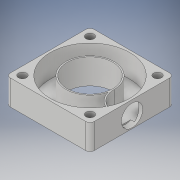
# Autodesk Inventor part: base3
Saved by Autodesk Inventor 2019 (Build 230136000, 136)
## iProperties
Created: 2020-10-29
Part Number: base3
Material: Genérico
Document SubType Name: Modeling
Designer: Juan M. Casillas
Density: 1 g/cm^3
Appearance: Valor por defecto
Author: Juan M. Casillas
## iProperties of the stored document base3_3DPrint.ipt
Created: 2020-10-29
Part Number: base3_3DPrint
Material: Genérico
Document SubType Name: Modeling
Designer: Juan M. Casillas
Density: 1 g/cm^3
Appearance: Valor por defecto
Author: Juan M. Casillas
Autodesk Inventor part; units mm, degrees
ref_plane "YZ Plane" through (0, 0, 0) normal (1, 0, 0) x (0, 1, 0)
ref_plane "XZ Plane" through (0, 0, 0) normal (0, 1, 0) x (-1, 0, 0)
ref_plane "XY Plane" through (0, 0, 0) normal (0, 0, 1) x (1, 0, 0)
sketch "Sketch1" plane through (0, 0, 0) normal (0, 1, 0) x (-1, 0, 0)
  line L0 (18, 20) -> (-18, 20)
  line L1 (-20, 18) -> (-20, -18)
  line L2 (-18, -20) -> (18, -20)
  line L3 (20, -18) -> (20, 18)
  line L4 (20, 20) -> (-20, -20) construction
  line L5 (-20, 20) -> (20, -20) construction
  circle A0 centre (0, 0) radius 11.5
  circle A1 centre (0, 0) radius 18.945
  arc A2 (20, 18) -> (18, 20) centre (18, 18) ccw
  arc A3 (18, -20) -> (20, -18) centre (18, -18) ccw
  arc A4 (-20, -18) -> (-18, -20) centre (-18, -18) ccw
  arc A5 (-18, 20) -> (-20, 18) centre (-18, 18) ccw
  dimension "d0" = 40
  dimension "d1" = 40
  dimension "d2" = 23
  dimension "d3" = 37.89
  dimension "d4" = 2
  constraints: 12 end point, 8 point on circle, 8 point on line, 8 tangent, 6 centre point, 3 equal radius, 2 coincident, 2 midpoint, 2 parallel, 1 horizontal, 1 perpendicular
  measures "d0" distance of L5.end L4.end
  measures "d1" distance of L4.end L5.start
  measures "d2" diameter of A0
  measures "d3" diameter of A1
  measures "d4" radius of A2
extrude "Extrusion1" add sketch "Sketch1" along normal blind 11
sketch "Sketch2" plane through (0, 0, 0) normal (0, -1, 0) x (1, 0, 0)
  line L0 (-20, -18) -> (-20, 18) projected
  arc A0 (-18, 20) -> (-20, 18) centre (-18, 18) ccw projected
  line L1 (-18, 20) -> (18, 20) projected
  arc A1 (20, 18) -> (18, 20) centre (18, 18) ccw projected
  line L2 (20, 18) -> (20, -18) projected
  arc A2 (18, -20) -> (20, -18) centre (18, -18) ccw projected
  line L3 (18, -20) -> (-18, -20) projected
  arc A3 (-20, -18) -> (-18, -20) centre (-18, -18) ccw projected
  point P0 (0, 0)
extrude "Extrusion2" add sketch "Sketch2" against normal blind 1
sketch "Sketch3" plane through (0, 11, 0) normal (0, 1, 0) x (1, 0, 0)
  circle A0 centre (0, 0) radius 11.5 projected
  circle A1 centre (0, 0) radius 10.9
  dimension "d9" = 0.6
  constraints: 1 centre point
  measures "d9" radial gap between concentric circles of A0 A1
extrude "Extrusion3" cut sketch "Sketch3" against normal through all contours A1
sketch "Sketch4" plane through (0, 11, 0) normal (0, 1, 0) x (1, 0, 0)
  circle A0 centre (0, 0) radius 18.945 construction
  line L0 (-18, -20) -> (18, -20) construction
  arc A1 (18, -20) -> (20, -18) centre (18, -18) ccw construction
  line L1 (20, -18) -> (20, 18) construction
  arc A2 (20, 18) -> (18, 20) centre (18, 18) ccw construction
  line L2 (18, 20) -> (-18, 20) construction
  arc A3 (-18, 20) -> (-20, 18) centre (-18, 18) ccw construction
  line L3 (-20, 18) -> (-20, -18) construction
  arc A4 (-20, -18) -> (-18, -20) centre (-18, -18) ccw construction
  line L4 (-16.1, -16.1) -> (16.1, -16.1) construction
  line L5 (16.1, -16.1) -> (16.1, 16.1) construction
  line L6 (16.1, 16.1) -> (-16.1, 16.1) construction
  line L7 (-16.1, 16.1) -> (-16.1, -16.1) construction
  line L8 (-16.1, -16.1) -> (16.1, 16.1) construction
  line L9 (16.1, -16.1) -> (-16.1, 16.1) construction
  point P0 (0, 0)
  dimension "d12" = 32.2
  dimension "d13" = 32.2
  constraints: 12 end point, 5 coincident, 3 midpoint, 2 parallel, 1 horizontal, 1 perpendicular
  measures "d12" distance of L6.end L5.end
  measures "d13" distance of L5.end L4.end
hole "Hole1" at (-16.1, 11, 16.1) at (-16.1, 11, -16.1) at (16.1, 11, -16.1) at (16.1, 11, 16.1) direction (0, -1, 0) diameter 3.85 depth 10
sketch "Sketch14" plane through (20, 0, -18) normal (1, 0, 0) x (0, 0, -1)
  line L0 (0, 0) -> (0, 11) construction
  line L1 (-36, 11) -> (0, 11) construction
  line L2 (-36, 0) -> (-36, 11) construction
  line L3 (-36, 0) -> (0, 0) construction
  line L4 (-25.5, 10) -> (-10.5, 10)
  line L5 (-10.5, 10) -> (-10.5, 1)
  line L6 (-10.5, 1) -> (-25.5, 1)
  line L7 (-25.5, 1) -> (-25.5, 10)
  line L8 (-25.5, 10) -> (-10.5, 1) construction
  line L9 (-10.5, 10) -> (-25.5, 1) construction
  point P0 (-18, 0)
  point P1 (-18, 5.5)
  dimension "d47" = 15
  dimension "d48" = 9
  constraints: 12 end point, 2 midpoint, 2 parallel, 1 horizontal, 1 perpendicular
  measures "d47" distance of L5.end L6.end
  measures "d48" distance of L4.end L5.end
extrude "Extrusion12" cut sketch "Sketch14" against normal blind 3
fillet "Fillet2" radius 2 2 edges at (17.3972, 5.5, 7.5) (17.3972, 5.5, -7.5)
sketch "Sketch15" plane through (0, 1, 0) normal (0, 1, 0) x (1, 0, 0)
  arc A0 (18.6666, -7.5) -> (16.8842, -8.5929) centre (18.6666, -9.5) ccw construction
  line L0 (20, -7.5) -> (18.6666, -7.5) construction
  line L1 (20, 7.5) -> (20, -7.5) construction
  line L2 (20, 7.5) -> (18.6666, 7.5) construction
  arc A1 (16.8842, 8.5929) -> (18.6666, 7.5) centre (18.6666, 9.5) ccw construction
  arc A2 (16.6035, -9.1235) -> (16.8842, -8.5929) centre (0, 0) ccw
  arc A3 (11.2223, -2.5118) -> (11.5, 0.0176) centre (0, 0) ccw
  arc A4 (11.5, 0.0176) -> (16.8842, -8.5929) centre (21.1006, 0.0323) ccw
  arc A5 (10.9, 0.0167) -> (16.6207, -9.1319) centre (21.1006, 0.0323) ccw
  dimension "d52" = 0.6
  constraints: 10 point on circle, 7 centre point, 1 tangent
  measures "d52" radial gap between concentric circles of A4 A5
extrude "Extrusion13" add sketch "Sketch15" along normal up to surface (10 mm away)
sketch "Sketch16" plane through (20, 10, -7.5) normal (0, -1, 0) x (1, 0, 0)
  arc A0 (-3.1158, -1.0929) -> (-3.1158, 16.0929) centre (-20, 7.5) ccw projected
  arc A1 (-1.3334, 0) -> (-3.1158, -1.0929) centre (-1.3334, -2) ccw projected
  line L0 (0, 0) -> (-1.3334, 0) projected
  line L1 (0, 15) -> (0, 0) projected
  line L2 (0, 15) -> (-1.3334, 15) projected
  arc A2 (-3.1158, 16.0929) -> (-1.3334, 15) centre (-1.3334, 17) ccw projected
extrude "Extrusion14" add sketch "Sketch16" along normal up to surface (9 mm away)
sketch "Sketch17" plane through (20, 0, -18) normal (1, 0, 0) x (0, 0, -1)
  line L0 (0, 0) -> (0, 11) construction
  line L1 (-36, 11) -> (0, 11) construction
  line L2 (-36, 0) -> (-36, 11) construction
  line L3 (-36, 0) -> (0, 0) construction
  circle A0 centre (-17.9824, 5.5) radius 5.1
  point P0 (-18, 0)
  dimension "d57" = 10.2
  constraints: 1 centre point
  measures "d57" diameter of A0
extrude "Extrusion15" cut sketch "Sketch17" against normal blind 3
sketch "Sketch18" plane through (0, 11, 0) normal (0, 1, 0) x (1, 0, 0)
  line L0 (-18, -20) -> (18, -20) projected
  arc A0 (18, -20) -> (20, -18) centre (18, -18) ccw projected
  line L1 (20, -18) -> (20, 18) projected
  arc A1 (20, 18) -> (18, 20) centre (18, 18) ccw projected
  line L2 (18, 20) -> (-18, 20) projected
  arc A2 (-18, 20) -> (-20, 18) centre (-18, 18) ccw projected
  line L3 (-20, 18) -> (-20, -18) projected
  arc A3 (-20, -18) -> (-18, -20) centre (-18, -18) ccw projected
  circle A4 centre (16.1, -16.1) radius 1.925 projected
  circle A5 centre (-16.1, 16.1) radius 1.925 projected
  circle A6 centre (-16.1, -16.1) radius 1.925 projected
  circle A7 centre (16.1, 16.1) radius 1.925 projected
  circle A8 centre (0, 0) radius 10.9 projected
  arc A9 (11.5, 0.0176) -> (11.2223, -2.5118) centre (0, 0) ccw projected
  arc A10 (11.2223, -2.5118) -> (16.6035, -9.1235) centre (21.1006, 0.0323) ccw projected
  arc A11 (16.8842, -8.5929) -> (16.6035, -9.1235) centre (0, 0) ccw projected
  arc A12 (11.5, 0.0176) -> (16.8842, -8.5929) centre (21.1006, 0.0323) ccw projected
extrude "Extrusion16" add sketch "Sketch18" along normal blind 1
sketch "Sketch5" plane through (20, 0, -18) normal (1, 0, 0) x (0, 0, -1)
  line L0 (0, 0) -> (0, 11) construction
  line L1 (-36, 11) -> (0, 11) construction
  line L2 (-36, 0) -> (-36, 11) construction
  line L3 (-36, 0) -> (0, 0) construction
  line L4 (-20.5, 10) -> (-5.5, 10)
  line L5 (-5.5, 10) -> (-5.5, 1)
  line L6 (-5.5, 1) -> (-20.5, 1)
  line L7 (-20.5, 1) -> (-20.5, 10)
  line L8 (-20.5, 10) -> (-5.5, 1) construction
  line L9 (-5.5, 10) -> (-20.5, 1) construction
  point P0 (-18, 0)
  point P1 (-13, 5.5)
  dimension "d21" = 15
  dimension "d22" = 9
  constraints: 12 end point, 2 midpoint, 2 parallel, 1 horizontal, 1 perpendicular
  measures "d21" distance of L5.end L6.end
  measures "d22" distance of L4.end L5.end
sketch "Sketch6" plane through (0, 1, 0) normal (0, 1, 0) x (1, 0, 0)
  line L0 (20, -2.5) -> (18.7339, -2.5) construction
  arc A0 (15.4996, 2.2947) -> (15.8884, 4.3911) centre (6.7587, 5) ccw
  arc A1 (15.8884, 4.3911) -> (18.7339, -2.5) centre (25.6093, 4.3721) ccw
  arc A2 (15.4996, 2.2947) -> (18.3979, -3.0115) centre (25.6093, 4.3721) ccw
  arc A3 (18.3979, -3.0115) -> (18.7339, -2.5) centre (6.7587, 5) ccw
  arc A4 (18.3979, -3.0115) -> (18.7339, -2.5) centre (6.7587, 5) ccw
  point P0 (0, 0)
  dimension "d25" = 0.6
  constraints: 11 point on circle, 6 centre point
  measures "d25" radial gap between concentric circles of A1 A2
sketch "Sketch12" plane through (20, 10, -12.5) normal (0, -1, 0) x (1, 0, 0)
  arc A0 (-4, 2.4397) -> (-1.2661, 15) centre (-20, 12.5) ccw projected
  line L0 (0, 0) -> (-4, 0) projected
  line L1 (0, 15) -> (0, 0) projected
  line L2 (0, 15) -> (-1.2661, 15) projected
  line L3 (-4, 2.4397) -> (-4, 0) projected
sketch "Sketch13" plane through (20, 0, -18) normal (1, 0, 0) x (0, 0, -1)
  line L0 (0, 0) -> (0, 11) construction
  line L1 (-36, 11) -> (0, 11) construction
  line L2 (-36, 0) -> (-36, 11) construction
  line L3 (-36, 0) -> (0, 0) construction
  circle A0 centre (-13, 5.5) radius 5.1
  point P0 (-18, 0)
  dimension "d44" = 10.2
  constraints: 1 centre point
  measures "d44" diameter of A0
sketch "Sketch8" plane through (20, 0, -13) normal (1, 0, 0) x (0, 0, -1)
  line L0 (-20.5, 10) -> (-5.5, 10) projected
  line L1 (-20.5, 1) -> (-20.5, 10) projected
  line L2 (-5.5, 1) -> (-20.5, 1) projected
  line L3 (-5.5, 10) -> (-5.5, 1) projected
  line L4 (-20.3, 9.8) -> (-5.7, 9.8)
  line L5 (-5.7, 9.8) -> (-5.7, 1.2)
  line L6 (-5.7, 1.2) -> (-20.3, 1.2)
  line L7 (-20.3, 1.2) -> (-20.3, 9.8)
  point P0 (-13, 0)
  dimension "d30" = 0.2
  dimension "d33" = 1
  dimension "d34" = 0.6
  constraints: 16 end point, 6 other
  measures "d33" distance between parallel lines of L1 L4
sketch "Sketch11" plane through (22.6, 0, -13) normal (1, 0, 0) x (0, 0, -1)
  line L0 (-21.3, 10.8) -> (-21.3, 0.2) construction
  line L1 (-21.3, 0.2) -> (-4.7, 0.2) construction
  line L2 (-4.7, 0.2) -> (-4.7, 10.8) construction
  line L3 (-4.7, 10.8) -> (-21.3, 10.8) construction
  circle A0 centre (-13, 5.5) radius 5.125
  point P0 (-13, 0)
  dimension "d39" = 10.25
  constraints: 1 centre point
  measures "d39" diameter of A0
body "Solid1"
